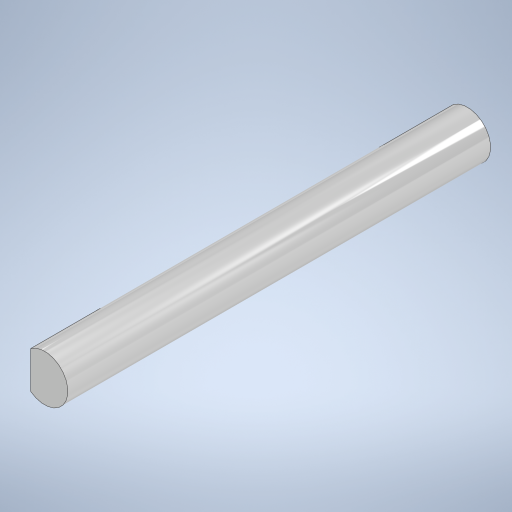
# Autodesk Inventor part: shaft
Saved by Autodesk Inventor 2024 (Build 280153000, 153)
## iProperties
Created: 2025-03-10
Part Number: shaft
Material: アルミニウム 5052 H32
Document SubType Name: Modeling
Designer: 1412z
Density: 2.68 g/cm^3
Appearance: アルミニウム - つや出し
Author: 1412z
Autodesk Inventor part; units mm, degrees
ref_plane "YZ Plane" through (0, 0, 0) normal (1, 0, 0) x (0, 1, 0)
ref_plane "XZ Plane" through (0, 0, 0) normal (0, 1, 0) x (-1, 0, 0)
ref_plane "XY Plane" through (0, 0, 0) normal (0, 0, 1) x (1, 0, 0)
sketch "スケッチ1" plane through (0, 0, 0) normal (0, 0, 1) x (1, 0, 0)
  circle A0 centre (0, 0) radius 2
  dimension "d0" = 4
  constraints: 1 centre point, 1 coincident
  measures "d0" diameter of A0
extrude "押し出し1" add sketch "スケッチ1" along normal blind 36.4
sketch "スケッチ2" plane through (0, 0, 36.4) normal (0, 0, 1) x (1, 0, 0)
  circle A0 centre (0, 0) radius 2 projected
  line L0 (-1.2, -1.6) -> (-1.2, 1.6)
  circle A1 centre (0, 0) radius 2 projected
  dimension "d4" = 3.2
  constraints: 2 end point, 2 point on circle, 1 vertical
  measures "d4" distance of L0.start L0.end
extrude "押し出し2" cut sketch "スケッチ2" against normal blind 6 contours L0 A0 picked at (-1.3118, -0.4272)
sketch "スケッチ3" plane through (0, 0, 0) normal (0, 0, -1) x (-1, 0, 0)
  line L0 (1.2, 1.6) -> (1.2, -1.6)
  circle A0 centre (0, 0) radius 2 projected
  dimension "d7" = 3.2
  constraints: 2 end point, 2 point on circle, 1 vertical
  measures "d7" distance of L0.start L0.end
extrude "押し出し3" cut sketch "スケッチ3" against normal blind 6 contours A0 L0 picked at (1.6903, 0)
